Autodesk Inventor part; units mm, degrees
(part 2 of 3)
  spline S290 degree 2 poles (47.4504, -3.8325) (47.4504, -4.6086) (47.1983, -5.9037) (46.9314, -6.3684) knots 0 0 0 1 2 2 2
  spline S291 degree 2 poles (46.9314, -6.3684) (46.6595, -6.838) (45.8438, -7.3422) (45.2506, -7.3422) knots 0 0 0 1 2 2 2
  spline S292 degree 2 poles (45.2506, -7.3422) (45.048, -7.3422) (44.613, -7.2681) (44.5438, -7.2384) knots 0 0 0 1 2 2 2
  line L295 (44.5438, -7.2384) -> (44.5438, -6.0421)
  line L296 (44.5438, -6.0421) -> (44.6278, -6.0421)
  spline S293 degree 2 poles (44.6278, -6.0421) (44.7069, -6.1015) (45.0035, -6.23) (45.2605, -6.23) knots 0 0 0 1 2 2 2
  spline S294 degree 2 poles (45.2605, -6.23) (45.4731, -6.23) (45.8587, -6.0718) (46.002, -5.8988) knots 0 0 0 1 2 2 2
  spline S295 degree 2 poles (46.002, -5.8988) (46.1454, -5.7159) (46.3431, -5.1771) (46.3777, -4.7717) knots 0 0 0 1 2 2 2
  spline S296 degree 2 poles (46.3777, -4.7717) (46.1454, -4.9744) (45.7549, -5.1919) (45.4632, -5.1919) knots 0 0 0 1 2 2 2
  spline S297 degree 2 poles (45.4632, -5.1919) (45.2408, -5.1919) (44.8354, -5.0238) (44.6723, -4.8459) knots 0 0 0 1 2 2 2
  spline S298 degree 2 poles (44.6723, -4.8459) (44.4498, -4.6036) (44.1928, -3.8276) (44.1928, -3.2146) knots 0 0 0 1 2 2 2
  spline S299 degree 2 poles (44.1928, -3.2146) (44.1928, -2.7351) (44.4202, -1.9293) (44.6278, -1.6327) knots 0 0 0 1 2 2 2
  spline S300 degree 2 poles (44.6278, -1.6327) (44.8354, -1.3361) (45.4335, -1) (45.8043, -1) knots 0 0 0 1 2 2 2
  spline S301 degree 2 poles (45.8043, -1) (46.175, -1) (46.7534, -1.2966) (46.961, -1.608) knots 0 0 0 1 2 2 2
  spline S302 degree 2 poles (46.961, -1.608) (47.2032, -1.9541) (47.4504, -3.0515) (47.4504, -3.8325) knots 0 0 0 1 2 2 2
  spline S303 degree 2 poles (46.3925, -3.6051) (46.3925, -3.1058) (46.2739, -2.4632) (46.1701, -2.2853) knots 0 0 0 1 2 2 2
  spline S304 degree 2 poles (46.1701, -2.2853) (46.0959, -2.1518) (45.9081, -2.0381) (45.7994, -2.0381) knots 0 0 0 1 2 2 2
  spline S305 degree 2 poles (45.7994, -2.0381) (45.7054, -2.0381) (45.5275, -2.1468) (45.4434, -2.2853) knots 0 0 0 1 2 2 2
  spline S306 degree 2 poles (45.4434, -2.2853) (45.3693, -2.4039) (45.2655, -2.8636) (45.2655, -3.1355) knots 0 0 0 1 2 2 2
  spline S307 degree 2 poles (45.2655, -3.1355) (45.2655, -3.4321) (45.3693, -3.8127) (45.4632, -3.9264) knots 0 0 0 1 2 2 2
  spline S308 degree 2 poles (45.4632, -3.9264) (45.5522, -4.0401) (45.7895, -4.1291) (45.9328, -4.1291) knots 0 0 0 1 2 2 2
  spline S309 degree 2 poles (45.9328, -4.1291) (46.0515, -4.1291) (46.3085, -4.0352) (46.3827, -3.9857) knots 0 0 0 1 2 2 2
  spline S310 degree 2 poles (46.3827, -3.9857) (46.3827, -3.9412) (46.3925, -3.7732) (46.3925, -3.6051) knots 0 0 0 1 2 2 2
  line L297 (43.6441, 12.8852) -> (40.8264, 12.8852)
  line L298 (40.8264, 12.8852) -> (40.8264, 13.948)
  line L299 (40.8264, 13.948) -> (41.7261, 13.948)
  line L300 (41.7261, 13.948) -> (41.7261, 17.1759)
  line L301 (41.7261, 17.1759) -> (40.8264, 17.1759)
  line L302 (40.8264, 17.1759) -> (40.8264, 18.1695)
  spline S311 degree 2 poles (40.8264, 18.1695) (41.0241, 18.1695) (41.4147, 18.2437) (41.5333, 18.3228) knots 0 0 0 1 2 2 2
  spline S312 degree 2 poles (41.5333, 18.3228) (41.6668, 18.4216) (41.82, 18.7528) (41.8299, 19) knots 0 0 0 1 2 2 2
  line L303 (41.8299, 19) -> (42.7642, 19)
  line L304 (42.7642, 19) -> (42.7642, 13.948)
  line L305 (42.7642, 13.948) -> (43.6441, 13.948)
  line L306 (43.6441, 13.948) -> (43.6441, 12.8852)
  line L307 (47.4702, 17.7741) -> (45.656, 12.8852)
  line L308 (45.656, 12.8852) -> (44.4647, 12.8852)
  line L309 (44.4647, 12.8852) -> (46.3678, 17.8334)
  line L310 (46.3678, 17.8334) -> (44.3361, 17.8334)
  line L311 (44.3361, 17.8334) -> (44.3361, 18.9852)
  line L312 (44.3361, 18.9852) -> (47.4702, 18.9852)
  line L313 (47.4702, 18.9852) -> (47.4702, 17.7741)
  line L314 (23.6441, 12.8852) -> (20.8264, 12.8852)
  line L315 (20.8264, 12.8852) -> (20.8264, 13.948)
  line L316 (20.8264, 13.948) -> (21.7261, 13.948)
  line L317 (21.7261, 13.948) -> (21.7261, 17.1759)
  line L318 (21.7261, 17.1759) -> (20.8264, 17.1759)
  line L319 (20.8264, 17.1759) -> (20.8264, 18.1695)
  spline S313 degree 2 poles (20.8264, 18.1695) (21.0241, 18.1695) (21.4147, 18.2437) (21.5333, 18.3228) knots 0 0 0 1 2 2 2
  spline S314 degree 2 poles (21.5333, 18.3228) (21.6668, 18.4216) (21.82, 18.7528) (21.8299, 19) knots 0 0 0 1 2 2 2
  line L320 (21.8299, 19) -> (22.7642, 19)
  line L321 (22.7642, 19) -> (22.7642, 13.948)
  line L322 (22.7642, 13.948) -> (23.6441, 13.948)
  line L323 (23.6441, 13.948) -> (23.6441, 12.8852)
  spline S315 degree 2 poles (27.4652, 14.9515) (27.4652, 14.472) (27.2378, 13.6613) (27.0154, 13.3696) knots 0 0 0 1 2 2 2
  spline S316 degree 2 poles (27.0154, 13.3696) (26.7929, 13.078) (26.175, 12.7566) (25.7252, 12.7566) knots 0 0 0 1 2 2 2
  spline S317 degree 2 poles (25.7252, 12.7566) (25.2506, 12.7616) (24.5685, 12.984) (24.346, 13.1274) knots 0 0 0 1 2 2 2
  line L324 (24.346, 13.1274) -> (24.346, 14.4571)
  line L325 (24.346, 14.4571) -> (24.4449, 14.4571)
  spline S318 degree 2 poles (24.4449, 14.4571) (24.524, 14.3929) (24.7217, 14.2248) (24.8848, 14.1358) knots 0 0 0 1 2 2 2
  spline S319 degree 2 poles (24.8848, 14.1358) (25.0381, 14.0518) (25.3495, 13.9381) (25.5423, 13.9381) knots 0 0 0 1 2 2 2
  spline S320 degree 2 poles (25.5423, 13.9381) (25.7104, 13.9381) (26.091, 14.0567) (26.2096, 14.2149) knots 0 0 0 1 2 2 2
  spline S321 degree 2 poles (26.2096, 14.2149) (26.2937, 14.3385) (26.3925, 14.64) (26.3925, 14.8921) knots 0 0 0 1 2 2 2
  spline S322 degree 2 poles (26.3925, 14.8921) (26.3925, 15.1096) (26.269, 15.4161) (26.1701, 15.51) knots 0 0 0 1 2 2 2
  spline S323 degree 2 poles (26.1701, 15.51) (26.0218, 15.6485) (25.6115, 15.7276) (25.4632, 15.7276) knots 0 0 0 1 2 2 2
  spline S324 degree 2 poles (25.4632, 15.7276) (25.2259, 15.7276) (24.786, 15.6188) (24.6229, 15.5595) knots 0 0 0 1 2 2 2
  line L326 (24.6229, 15.5595) -> (24.5289, 15.5595)
  line L327 (24.5289, 15.5595) -> (24.5289, 18.9852)
  line L328 (24.5289, 18.9852) -> (27.3466, 18.9852)
  line L329 (27.3466, 18.9852) -> (27.3466, 17.8334)
  line L330 (27.3466, 17.8334) -> (25.5374, 17.8334)
  line L331 (25.5374, 17.8334) -> (25.5374, 16.82)
  spline S325 degree 2 poles (25.5374, 16.82) (25.6214, 16.8299) (25.8587, 16.8398) (25.9279, 16.8398) knots 0 0 0 1 2 2 2
  spline S326 degree 2 poles (25.9279, 16.8398) (26.2344, 16.8398) (26.7534, 16.6618) (26.9511, 16.4789) knots 0 0 0 1 2 2 2
  spline S327 degree 2 poles (26.9511, 16.4789) (27.1983, 16.2515) (27.4652, 15.4952) (27.4652, 14.9515) knots 0 0 0 1 2 2 2
  line L332 (33.6441, 12.7863) -> (30.8264, 12.7863)
  line L333 (30.8264, 12.7863) -> (30.8264, 13.8491)
  line L334 (30.8264, 13.8491) -> (31.7261, 13.8491)
  line L335 (31.7261, 13.8491) -> (31.7261, 17.0771)
  line L336 (31.7261, 17.0771) -> (30.8264, 17.0771)
  line L337 (30.8264, 17.0771) -> (30.8264, 18.0707)
  spline S328 degree 2 poles (30.8264, 18.0707) (31.0241, 18.0707) (31.4147, 18.1448) (31.5333, 18.2239) knots 0 0 0 1 2 2 2
  spline S329 degree 2 poles (31.5333, 18.2239) (31.6668, 18.3228) (31.82, 18.654) (31.8299, 18.9011) knots 0 0 0 1 2 2 2
  line L338 (31.8299, 18.9011) -> (32.7642, 18.9011)
  line L339 (32.7642, 18.9011) -> (32.7642, 13.8491)
  line L340 (32.7642, 13.8491) -> (33.6441, 13.8491)
  line L341 (33.6441, 13.8491) -> (33.6441, 12.7863)
  spline S330 degree 2 poles (37.5394, 14.8625) (37.5394, 13.8985) (36.6842, 12.6578) (35.9427, 12.6578) knots 0 0 0 1 2 2 2
  spline S331 degree 2 poles (35.9427, 12.6578) (35.572, 12.6578) (34.9837, 12.9643) (34.781, 13.2658) knots 0 0 0 1 2 2 2
  spline S332 degree 2 poles (34.781, 13.2658) (34.5388, 13.6168) (34.2818, 14.729) (34.2818, 15.5051) knots 0 0 0 1 2 2 2
  spline S333 degree 2 poles (34.2818, 15.5051) (34.2818, 16.3059) (34.524, 17.5516) (34.7959, 18.0311) knots 0 0 0 1 2 2 2
  spline S334 degree 2 poles (34.7959, 18.0311) (35.0529, 18.4859) (35.8982, 19) (36.4716, 19) knots 0 0 0 1 2 2 2
  spline S335 degree 2 poles (36.4716, 19) (36.6793, 19) (37.0994, 18.9209) (37.1785, 18.8962) knots 0 0 0 1 2 2 2
  line L342 (37.1785, 18.8962) -> (37.1785, 17.6999)
  line L343 (37.1785, 17.6999) -> (37.0994, 17.6999)
  spline S336 degree 2 poles (37.0994, 17.6999) (37.0253, 17.7543) (36.6842, 17.8878) (36.4618, 17.8878) knots 0 0 0 1 2 2 2
  spline S337 degree 2 poles (36.4618, 17.8878) (35.9625, 17.8878) (35.4187, 17.1314) (35.3545, 16.4295) knots 0 0 0 1 2 2 2
  spline S338 degree 2 poles (35.3545, 16.4295) (35.567, 16.6223) (35.9971, 16.8497) (36.269, 16.8497) knots 0 0 0 1 2 2 2
  spline S339 degree 2 poles (36.269, 16.8497) (36.4964, 16.8497) (36.9017, 16.6717) (37.0599, 16.5036) knots 0 0 0 1 2 2 2
  spline S340 degree 2 poles (37.0599, 16.5036) (37.2774, 16.2614) (37.5394, 15.4754) (37.5394, 14.8625) knots 0 0 0 1 2 2 2
  spline S341 degree 2 poles (36.2937, 13.943) (36.3777, 14.0913) (36.4667, 14.4374) (36.4667, 14.7883) knots 0 0 0 1 2 2 2
  spline S342 degree 2 poles (36.4667, 14.7883) (36.4667, 15.0849) (36.3629, 15.4705) (36.269, 15.5842) knots 0 0 0 1 2 2 2
  spline S343 degree 2 poles (36.269, 15.5842) (36.175, 15.7028) (35.9378, 15.7869) (35.7994, 15.7869) knots 0 0 0 1 2 2 2
  spline S344 degree 2 poles (35.7994, 15.7869) (35.6906, 15.7869) (35.4533, 15.7028) (35.3495, 15.6435) knots 0 0 0 1 2 2 2
  spline S345 degree 2 poles (35.3495, 15.6435) (35.3495, 15.604) (35.3446, 15.4161) (35.3446, 15.2728) knots 0 0 0 1 2 2 2
  spline S346 degree 2 poles (35.3446, 15.2728) (35.3446, 14.7438) (35.4731, 14.1062) (35.572, 13.943) knots 0 0 0 1 2 2 2
  spline S347 degree 2 poles (35.572, 13.943) (35.6461, 13.8096) (35.834, 13.6959) (35.9427, 13.6959) knots 0 0 0 1 2 2 2
  spline S348 degree 2 poles (35.9427, 13.6959) (36.0267, 13.6959) (36.2245, 13.8194) (36.2937, 13.943) knots 0 0 0 1 2 2 2
  line L344 (23.8319, -7.2186) -> (20.6979, -7.2186)
  line L345 (20.6979, -7.2186) -> (20.6979, -6.225)
  spline S349 degree 2 poles (20.6979, -6.225) (21.0983, -5.7703) (21.7261, -4.9694) (21.9683, -4.6086) knots 0 0 0 1 2 2 2
  spline S350 degree 2 poles (21.9683, -4.6086) (22.2797, -4.139) (22.5615, -3.4222) (22.5615, -3.0465) knots 0 0 0 1 2 2 2
  spline S351 degree 2 poles (22.5615, -3.0465) (22.5615, -2.6214) (22.2056, -2.1666) (21.8892, -2.1666) knots 0 0 0 1 2 2 2
  spline S352 degree 2 poles (21.8892, -2.1666) (21.7261, -2.1666) (21.4394, -2.2803) (21.2861, -2.3693) knots 0 0 0 1 2 2 2
  spline S353 degree 2 poles (21.2861, -2.3693) (21.1428, -2.4632) (20.9352, -2.6609) (20.8857, -2.7104) knots 0 0 0 1 2 2 2
  line L346 (20.8857, -2.7104) -> (20.8017, -2.7104)
  line L347 (20.8017, -2.7104) -> (20.8017, -1.3806)
  spline S354 degree 2 poles (20.8017, -1.3806) (20.9797, -1.257) (21.7508, -1) (22.1018, -1) knots 0 0 0 1 2 2 2
  spline S355 degree 2 poles (22.1018, -1) (22.863, -1) (23.6441, -1.9689) (23.6441, -2.8438) knots 0 0 0 1 2 2 2
  spline S356 degree 2 poles (23.6441, -2.8438) (23.6441, -3.3827) (23.2882, -4.4207) (22.8779, -5.0139) knots 0 0 0 1 2 2 2
  spline S357 degree 2 poles (22.8779, -5.0139) (22.6208, -5.3797) (22.1314, -5.9482) (22.0227, -6.0669) knots 0 0 0 1 2 2 2
  line L348 (22.0227, -6.0669) -> (23.8319, -6.0669)
  line L349 (23.8319, -6.0669) -> (23.8319, -7.2186)
  line L350 (27.4702, -2.3297) -> (25.656, -7.2186)
  line L351 (25.656, -7.2186) -> (24.4647, -7.2186)
  line L352 (24.4647, -7.2186) -> (26.3678, -2.2704)
  line L353 (26.3678, -2.2704) -> (24.3361, -2.2704)
  line L354 (24.3361, -2.2704) -> (24.3361, -1.1186)
  line L355 (24.3361, -1.1186) -> (27.4702, -1.1186)
  line L356 (27.4702, -1.1186) -> (27.4702, -2.3297)
  line L357 (23.8319, 2.7814) -> (20.6979, 2.7814)
  line L358 (20.6979, 2.7814) -> (20.6979, 3.775)
  spline S358 degree 2 poles (20.6979, 3.775) (21.0983, 4.2297) (21.7261, 5.0306) (21.9683, 5.3914) knots 0 0 0 1 2 2 2
  spline S359 degree 2 poles (21.9683, 5.3914) (22.2797, 5.861) (22.5615, 6.5778) (22.5615, 6.9535) knots 0 0 0 1 2 2 2
  spline S360 degree 2 poles (22.5615, 6.9535) (22.5615, 7.3786) (22.2056, 7.8334) (21.8892, 7.8334) knots 0 0 0 1 2 2 2
  spline S361 degree 2 poles (21.8892, 7.8334) (21.7261, 7.8334) (21.4394, 7.7197) (21.2861, 7.6307) knots 0 0 0 1 2 2 2
  spline S362 degree 2 poles (21.2861, 7.6307) (21.1428, 7.5368) (20.9352, 7.3391) (20.8857, 7.2896) knots 0 0 0 1 2 2 2
  line L359 (20.8857, 7.2896) -> (20.8017, 7.2896)
  line L360 (20.8017, 7.2896) -> (20.8017, 8.6194)
  spline S363 degree 2 poles (20.8017, 8.6194) (20.9797, 8.743) (21.7508, 9) (22.1018, 9) knots 0 0 0 1 2 2 2
  spline S364 degree 2 poles (22.1018, 9) (22.863, 9) (23.6441, 8.0311) (23.6441, 7.1562) knots 0 0 0 1 2 2 2
  spline S365 degree 2 poles (23.6441, 7.1562) (23.6441, 6.6173) (23.2882, 5.5793) (22.8779, 4.9861) knots 0 0 0 1 2 2 2
  spline S366 degree 2 poles (22.8779, 4.9861) (22.6208, 4.6203) (22.1314, 4.0518) (22.0227, 3.9331) knots 0 0 0 1 2 2 2
  line L361 (22.0227, 3.9331) -> (23.8319, 3.9331)
  line L362 (23.8319, 3.9331) -> (23.8319, 2.7814)
  line L363 (27.3763, 2.7814) -> (24.5586, 2.7814)
  line L364 (24.5586, 2.7814) -> (24.5586, 3.8442)
  line L365 (24.5586, 3.8442) -> (25.4583, 3.8442)
  line L366 (25.4583, 3.8442) -> (25.4583, 7.0721)
  line L367 (25.4583, 7.0721) -> (24.5586, 7.0721)
  line L368 (24.5586, 7.0721) -> (24.5586, 8.0657)
  spline S367 degree 2 poles (24.5586, 8.0657) (24.7563, 8.0657) (25.1468, 8.1399) (25.2655, 8.219) knots 0 0 0 1 2 2 2
  spline S368 degree 2 poles (25.2655, 8.219) (25.3989, 8.3178) (25.5522, 8.649) (25.5621, 8.8962) knots 0 0 0 1 2 2 2
  line L369 (25.5621, 8.8962) -> (26.4964, 8.8962)
  line L370 (26.4964, 8.8962) -> (26.4964, 3.8442)
  line L371 (26.4964, 3.8442) -> (27.3763, 3.8442)
  line L372 (27.3763, 3.8442) -> (27.3763, 2.7814)
  line L373 (53.8319, 2.7814) -> (50.6979, 2.7814)
  line L374 (50.6979, 2.7814) -> (50.6979, 3.775)
  spline S369 degree 2 poles (50.6979, 3.775) (51.0983, 4.2297) (51.7261, 5.0306) (51.9683, 5.3914) knots 0 0 0 1 2 2 2
  spline S370 degree 2 poles (51.9683, 5.3914) (52.2797, 5.861) (52.5615, 6.5778) (52.5615, 6.9535) knots 0 0 0 1 2 2 2
  spline S371 degree 2 poles (52.5615, 6.9535) (52.5615, 7.3786) (52.2056, 7.8334) (51.8892, 7.8334) knots 0 0 0 1 2 2 2
  spline S372 degree 2 poles (51.8892, 7.8334) (51.7261, 7.8334) (51.4394, 7.7197) (51.2861, 7.6307) knots 0 0 0 1 2 2 2
  spline S373 degree 2 poles (51.2861, 7.6307) (51.1428, 7.5368) (50.9352, 7.3391) (50.8857, 7.2896) knots 0 0 0 1 2 2 2
  line L375 (50.8857, 7.2896) -> (50.8017, 7.2896)
  line L376 (50.8017, 7.2896) -> (50.8017, 8.6194)
  spline S374 degree 2 poles (50.8017, 8.6194) (50.9797, 8.743) (51.7508, 9) (52.1018, 9) knots 0 0 0 1 2 2 2
  spline S375 degree 2 poles (52.1018, 9) (52.863, 9) (53.6441, 8.0311) (53.6441, 7.1562) knots 0 0 0 1 2 2 2
  spline S376 degree 2 poles (53.6441, 7.1562) (53.6441, 6.6173) (53.2882, 5.5793) (52.8779, 4.9861) knots 0 0 0 1 2 2 2
  spline S377 degree 2 poles (52.8779, 4.9861) (52.6208, 4.6203) (52.1314, 4.0518) (52.0227, 3.9331) knots 0 0 0 1 2 2 2
  line L377 (52.0227, 3.9331) -> (53.8319, 3.9331)
  line L378 (53.8319, 3.9331) -> (53.8319, 2.7814)
  line L379 (57.6086, 4.205) -> (57.0352, 4.205)
  line L380 (57.0352, 4.205) -> (57.0352, 2.7665)
  line L381 (57.0352, 2.7665) -> (55.9971, 2.7665)
  line L382 (55.9971, 2.7665) -> (55.9971, 4.205)
  line L383 (55.9971, 4.205) -> (54.1285, 4.205)
  line L384 (54.1285, 4.205) -> (54.1285, 5.342)
  line L385 (54.1285, 5.342) -> (55.9625, 8.8814)
  line L386 (55.9625, 8.8814) -> (57.0352, 8.8814)
  line L387 (57.0352, 8.8814) -> (57.0352, 5.3024)
  line L388 (57.0352, 5.3024) -> (57.6086, 5.3024)
  line L389 (57.6086, 5.3024) -> (57.6086, 4.205)
  line L390 (55.9971, 5.3024) -> (55.9971, 7.3737)
  line L391 (55.9971, 7.3737) -> (54.9244, 5.3024)
  line L392 (54.9244, 5.3024) -> (55.9971, 5.3024)
  line L393 (43.8319, 2.7715) -> (40.6979, 2.7715)
  line L394 (40.6979, 2.7715) -> (40.6979, 3.7651)
  spline S378 degree 2 poles (40.6979, 3.7651) (41.0983, 4.2199) (41.7261, 5.0207) (41.9683, 5.3815) knots 0 0 0 1 2 2 2
  spline S379 degree 2 poles (41.9683, 5.3815) (42.2797, 5.8511) (42.5615, 6.5679) (42.5615, 6.9436) knots 0 0 0 1 2 2 2
  spline S380 degree 2 poles (42.5615, 6.9436) (42.5615, 7.3687) (42.2056, 7.8235) (41.8892, 7.8235) knots 0 0 0 1 2 2 2
  spline S381 degree 2 poles (41.8892, 7.8235) (41.7261, 7.8235) (41.4394, 7.7098) (41.2861, 7.6208) knots 0 0 0 1 2 2 2
  spline S382 degree 2 poles (41.2861, 7.6208) (41.1428, 7.5269) (40.9352, 7.3292) (40.8857, 7.2797) knots 0 0 0 1 2 2 2
  line L395 (40.8857, 7.2797) -> (40.8017, 7.2797)
  line L396 (40.8017, 7.2797) -> (40.8017, 8.6095)
  spline S383 degree 2 poles (40.8017, 8.6095) (40.9797, 8.7331) (41.7508, 8.9901) (42.1018, 8.9901) knots 0 0 0 1 2 2 2
  spline S384 degree 2 poles (42.1018, 8.9901) (42.863, 8.9901) (43.6441, 8.0212) (43.6441, 7.1463) knots 0 0 0 1 2 2 2
  spline S385 degree 2 poles (43.6441, 7.1463) (43.6441, 6.6075) (43.2882, 5.5694) (42.8779, 4.9762) knots 0 0 0 1 2 2 2
  spline S386 degree 2 poles (42.8779, 4.9762) (42.6208, 4.6104) (42.1314, 4.0419) (42.0227, 3.9233) knots 0 0 0 1 2 2 2
  line L397 (42.0227, 3.9233) -> (43.8319, 3.9233)
  line L398 (43.8319, 3.9233) -> (43.8319, 2.7715)
  spline S387 degree 2 poles (47.4553, 4.6203) (47.4553, 4.1704) (47.223, 3.4339) (47.0006, 3.1768) knots 0 0 0 1 2 2 2
  spline S388 degree 2 poles (47.0006, 3.1768) (46.7732, 2.9198) (46.1652, 2.6429) (45.7301, 2.6429) knots 0 0 0 1 2 2 2
  spline S389 degree 2 poles (45.7301, 2.6429) (45.2309, 2.6429) (44.519, 2.8802) (44.2966, 3.0285) knots 0 0 0 1 2 2 2
  line L399 (44.2966, 3.0285) -> (44.2966, 4.3533)
  line L400 (44.2966, 4.3533) -> (44.4004, 4.3533)
  spline S390 degree 2 poles (44.4004, 4.3533) (44.6327, 4.1408) (45.2655, 3.8244) (45.5275, 3.8244) knots 0 0 0 1 2 2 2
  spline S391 degree 2 poles (45.5275, 3.8244) (45.6807, 3.8244) (46.0465, 3.9035) (46.1701, 4.032) knots 0 0 0 1 2 2 2
  spline S392 degree 2 poles (46.1701, 4.032) (46.264, 4.1358) (46.3827, 4.4374) (46.3827, 4.7092) knots 0 0 0 1 2 2 2
  spline S393 degree 2 poles (46.3827, 4.7092) (46.3827, 4.9811) (46.2146, 5.2728) (46.0811, 5.342) knots 0 0 0 1 2 2 2
  spline S394 degree 2 poles (46.0811, 5.342) (45.9427, 5.4112) (45.5571, 5.426) (45.4138, 5.426) knots 0 0 0 1 2 2 2
  line L401 (45.4138, 5.426) -> (45.2309, 5.426)
  line L402 (45.2309, 5.426) -> (45.2309, 6.4987)
  line L403 (45.2309, 6.4987) -> (45.3989, 6.4987)
  spline S395 degree 2 poles (45.3989, 6.4987) (45.5917, 6.4987) (45.913, 6.5481) (46.0267, 6.6223) knots 0 0 0 1 2 2 2
  spline S396 degree 2 poles (46.0267, 6.6223) (46.1404, 6.7014) (46.269, 6.9782) (46.269, 7.2155) knots 0 0 0 1 2 2 2
  spline S397 degree 2 poles (46.269, 7.2155) (46.269, 7.4033) (46.1503, 7.6357) (46.0613, 7.6999) knots 0 0 0 1 2 2 2
  spline S398 degree 2 poles (46.0613, 7.6999) (45.9575, 7.7741) (45.6857, 7.8235) (45.5868, 7.8235) knots 0 0 0 1 2 2 2
  spline S399 degree 2 poles (45.5868, 7.8235) (45.4335, 7.8235) (45.1073, 7.7197) (44.9541, 7.6357) knots 0 0 0 1 2 2 2
  spline S400 degree 2 poles (44.9541, 7.6357) (44.8354, 7.5714) (44.5734, 7.3638) (44.5092, 7.3094) knots 0 0 0 1 2 2 2
  line L404 (44.5092, 7.3094) -> (44.4202, 7.3094)
  line L405 (44.4202, 7.3094) -> (44.4202, 8.6144)
  spline S401 degree 2 poles (44.4202, 8.6144) (44.6377, 8.7479) (45.3841, 9) (45.7746, 9) knots 0 0 0 1 2 2 2
  spline S402 degree 2 poles (45.7746, 9) (46.1553, 9) (46.7089, 8.8122) (46.9066, 8.6293) knots 0 0 0 1 2 2 2
  spline S403 degree 2 poles (46.9066, 8.6293) (47.1241, 8.4365) (47.3417, 7.8433) (47.3417, 7.4725) knots 0 0 0 1 2 2 2
  spline S404 degree 2 poles (47.3417, 7.4725) (47.3417, 6.9485) (46.9215, 6.1675) (46.5804, 6.0538) knots 0 0 0 1 2 2 2
  line L406 (46.5804, 6.0538) -> (46.5804, 5.9945)
  spline S405 degree 2 poles (46.5804, 5.9945) (46.7336, 5.9648) (47.0203, 5.8066) (47.1588, 5.6287) knots 0 0 0 1 2 2 2
  spline S406 degree 2 poles (47.1588, 5.6287) (47.2873, 5.4705) (47.4553, 4.9663) (47.4553, 4.6203) knots 0 0 0 1 2 2 2
  line L407 (53.6441, 12.7616) -> (50.8264, 12.7616)
  line L408 (50.8264, 12.7616) -> (50.8264, 13.8244)
  line L409 (50.8264, 13.8244) -> (51.7261, 13.8244)
  line L410 (51.7261, 13.8244) -> (51.7261, 17.0524)
  line L411 (51.7261, 17.0524) -> (50.8264, 17.0524)
  line L412 (50.8264, 17.0524) -> (50.8264, 18.0459)
  spline S407 degree 2 poles (50.8264, 18.0459) (51.0241, 18.0459) (51.4147, 18.1201) (51.5333, 18.1992) knots 0 0 0 1 2 2 2
  spline S408 degree 2 poles (51.5333, 18.1992) (51.6668, 18.2981) (51.82, 18.6293) (51.8299, 18.8764) knots 0 0 0 1 2 2 2
  line L413 (51.8299, 18.8764) -> (52.7642, 18.8764)
  line L414 (52.7642, 18.8764) -> (52.7642, 13.8244)
  line L415 (52.7642, 13.8244) -> (53.6441, 13.8244)
  line L416 (53.6441, 13.8244) -> (53.6441, 12.7616)
  spline S409 degree 2 poles (57.5542, 14.4571) (57.5542, 14.0666) (57.3268, 13.3894) (57.1093, 13.1422) knots 0 0 0 1 2 2 2
  spline S410 degree 2 poles (57.1093, 13.1422) (56.8918, 12.8951) (56.264, 12.6182) (55.8587, 12.6182) knots 0 0 0 1 2 2 2
  spline S411 degree 2 poles (55.8587, 12.6182) (55.4286, 12.6182) (54.781, 12.9) (54.5784, 13.1422) knots 0 0 0 1 2 2 2
  spline S412 degree 2 poles (54.5784, 13.1422) (54.3707, 13.3844) (54.178, 14.0419) (54.178, 14.4077) knots 0 0 0 1 2 2 2
  spline S413 degree 2 poles (54.178, 14.4077) (54.178, 14.9317) (54.5833, 15.6287) (54.9639, 15.861) knots 0 0 0 1 2 2 2
  line L417 (54.9639, 15.861) -> (54.9639, 15.8857)
  spline S414 degree 2 poles (54.9639, 15.8857) (54.5882, 16.1477) (54.2917, 16.8942) (54.2917, 17.3539) knots 0 0 0 1 2 2 2
  spline S415 degree 2 poles (54.2917, 17.3539) (54.2917, 17.69) (54.4993, 18.2783) (54.7069, 18.5106) knots 0 0 0 1 2 2 2
  spline S416 degree 2 poles (54.7069, 18.5106) (54.8997, 18.7331) (55.4978, 19) (55.8735, 19) knots 0 0 0 1 2 2 2
  spline S417 degree 2 poles (55.8735, 19) (56.269, 19) (56.8572, 18.7578) (57.0451, 18.56) knots 0 0 0 1 2 2 2
  spline S418 degree 2 poles (57.0451, 18.56) (57.2378, 18.3623) (57.4455, 17.7889) (57.4455, 17.4577) knots 0 0 0 1 2 2 2
  spline S419 degree 2 poles (57.4455, 17.4577) (57.4455, 17.0227) (57.0945, 16.3257) (56.7287, 16.0835) knots 0 0 0 1 2 2 2
  line L418 (56.7287, 16.0835) -> (56.7287, 16.0637)
  spline S420 degree 2 poles (56.7287, 16.0637) (57.1538, 15.8165) (57.5542, 15.0157) (57.5542, 14.4571) knots 0 0 0 1 2 2 2
  spline S421 degree 2 poles (56.4964, 14.3929) (56.4964, 14.6944) (56.3184, 15.0108) (56.0218, 15.2135) knots 0 0 0 1 2 2 2
  spline S422 degree 2 poles (56.0218, 15.2135) (55.9378, 15.2678) (55.6263, 15.4408) (55.5028, 15.515) knots 0 0 0 1 2 2 2
  spline S423 degree 2 poles (55.5028, 15.515) (55.394, 15.3568) (55.216, 14.8823) (55.216, 14.6005) knots 0 0 0 1 2 2 2
  spline S424 degree 2 poles (55.216, 14.6005) (55.216, 14.1754) (55.5967, 13.6662) (55.9081, 13.6662) knots 0 0 0 1 2 2 2
  spline S425 degree 2 poles (55.9081, 13.6662) (55.9921, 13.6662) (56.2096, 13.7453) (56.2937, 13.8244) knots 0 0 0 1 2 2 2
  spline S426 degree 2 poles (56.2937, 13.8244) (56.3827, 13.9183) (56.4964, 14.1754) (56.4964, 14.3929) knots 0 0 0 1 2 2 2
  spline S427 degree 2 poles (56.4074, 17.2797) (56.4074, 17.5912) (56.1207, 17.9619) (55.8735, 17.9619) knots 0 0 0 1 2 2 2
  spline S428 degree 2 poles (55.8735, 17.9619) (55.6412, 17.9619) (55.3495, 17.6258) (55.3495, 17.3786) knots 0 0 0 1 2 2 2
  spline S429 degree 2 poles (55.3495, 17.3786) (55.3495, 17.1364) (55.5225, 16.8348) (55.7104, 16.7113) knots 0 0 0 1 2 2 2
  spline S430 degree 2 poles (55.7104, 16.7113) (55.7895, 16.6519) (56.007, 16.5284) (56.1948, 16.4295) knots 0 0 0 1 2 2 2
  spline S431 degree 2 poles (56.1948, 16.4295) (56.3036, 16.6371) (56.4074, 17.0276) (56.4074, 17.2797) knots 0 0 0 1 2 2 2
  line L419 (33.8319, -7.2384) -> (30.6979, -7.2384)
  line L420 (30.6979, -7.2384) -> (30.6979, -6.2448)
  spline S432 degree 2 poles (30.6979, -6.2448) (31.0983, -5.79) (31.7261, -4.9892) (31.9683, -4.6284) knots 0 0 0 1 2 2 2
  spline S433 degree 2 poles (31.9683, -4.6284) (32.2797, -4.1588) (32.5615, -3.442) (32.5615, -3.0663) knots 0 0 0 1 2 2 2
  spline S434 degree 2 poles (32.5615, -3.0663) (32.5615, -2.6412) (32.2056, -2.1864) (31.8892, -2.1864) knots 0 0 0 1 2 2 2
  spline S435 degree 2 poles (31.8892, -2.1864) (31.7261, -2.1864) (31.4394, -2.3001) (31.2861, -2.3891) knots 0 0 0 1 2 2 2
  spline S436 degree 2 poles (31.2861, -2.3891) (31.1428, -2.483) (30.9352, -2.6807) (30.8857, -2.7301) knots 0 0 0 1 2 2 2
  line L421 (30.8857, -2.7301) -> (30.8017, -2.7301)
  line L422 (30.8017, -2.7301) -> (30.8017, -1.4004)
  spline S437 degree 2 poles (30.8017, -1.4004) (30.9797, -1.2768) (31.7508, -1.0198) (32.1018, -1.0198) knots 0 0 0 1 2 2 2
  spline S438 degree 2 poles (32.1018, -1.0198) (32.863, -1.0198) (33.6441, -1.9887) (33.6441, -2.8636) knots 0 0 0 1 2 2 2
  spline S439 degree 2 poles (33.6441, -2.8636) (33.6441, -3.4024) (33.2882, -4.4405) (32.8779, -5.0337) knots 0 0 0 1 2 2 2
  spline S440 degree 2 poles (32.8779, -5.0337) (32.6208, -5.3995) (32.1314, -5.968) (32.0227, -6.0866) knots 0 0 0 1 2 2 2
  line L423 (32.0227, -6.0866) -> (33.8319, -6.0866)
  line L424 (33.8319, -6.0866) -> (33.8319, -7.2384)
  spline S441 degree 2 poles (37.5542, -5.5429) (37.5542, -5.9334) (37.3268, -6.6106) (37.1093, -6.8578) knots 0 0 0 1 2 2 2
  spline S442 degree 2 poles (37.1093, -6.8578) (36.8918, -7.1049) (36.264, -7.3818) (35.8587, -7.3818) knots 0 0 0 1 2 2 2
  spline S443 degree 2 poles (35.8587, -7.3818) (35.4286, -7.3818) (34.781, -7.1) (34.5784, -6.8578) knots 0 0 0 1 2 2 2
  spline S444 degree 2 poles (34.5784, -6.8578) (34.3707, -6.6156) (34.178, -5.9581) (34.178, -5.5923) knots 0 0 0 1 2 2 2
  spline S445 degree 2 poles (34.178, -5.5923) (34.178, -5.0683) (34.5833, -4.3713) (34.9639, -4.139) knots 0 0 0 1 2 2 2
  line L425 (34.9639, -4.139) -> (34.9639, -4.1143)
  spline S446 degree 2 poles (34.9639, -4.1143) (34.5882, -3.8523) (34.2917, -3.1058) (34.2917, -2.6461) knots 0 0 0 1 2 2 2
  spline S447 degree 2 poles (34.2917, -2.6461) (34.2917, -2.31) (34.4993, -1.7217) (34.7069, -1.4894) knots 0 0 0 1 2 2 2
  spline S448 degree 2 poles (34.7069, -1.4894) (34.8997, -1.2669) (35.4978, -1) (35.8735, -1) knots 0 0 0 1 2 2 2
  spline S449 degree 2 poles (35.8735, -1) (36.269, -1) (36.8572, -1.2422) (37.0451, -1.44) knots 0 0 0 1 2 2 2
  spline S450 degree 2 poles (37.0451, -1.44) (37.2378, -1.6377) (37.4455, -2.2111) (37.4455, -2.5423) knots 0 0 0 1 2 2 2
  spline S451 degree 2 poles (37.4455, -2.5423) (37.4455, -2.9773) (37.0945, -3.6743) (36.7287, -3.9165) knots 0 0 0 1 2 2 2
  line L426 (36.7287, -3.9165) -> (36.7287, -3.9363)
  spline S452 degree 2 poles (36.7287, -3.9363) (37.1538, -4.1835) (37.5542, -4.9843) (37.5542, -5.5429) knots 0 0 0 1 2 2 2
  spline S453 degree 2 poles (36.4964, -5.6071) (36.4964, -5.3056) (36.3184, -4.9892) (36.0218, -4.7865) knots 0 0 0 1 2 2 2
  spline S454 degree 2 poles (36.0218, -4.7865) (35.9378, -4.7322) (35.6263, -4.5592) (35.5028, -4.485) knots 0 0 0 1 2 2 2
  spline S455 degree 2 poles (35.5028, -4.485) (35.394, -4.6432) (35.216, -5.1177) (35.216, -5.3995) knots 0 0 0 1 2 2 2
  spline S456 degree 2 poles (35.216, -5.3995) (35.216, -5.8246) (35.5967, -6.3338) (35.9081, -6.3338) knots 0 0 0 1 2 2 2
  spline S457 degree 2 poles (35.9081, -6.3338) (35.9921, -6.3338) (36.2096, -6.2547) (36.2937, -6.1756) knots 0 0 0 1 2 2 2
  spline S458 degree 2 poles (36.2937, -6.1756) (36.3827, -6.0817) (36.4964, -5.8246) (36.4964, -5.6071) knots 0 0 0 1 2 2 2
  spline S459 degree 2 poles (36.4074, -2.7203) (36.4074, -2.4088) (36.1207, -2.0381) (35.8735, -2.0381) knots 0 0 0 1 2 2 2
  spline S460 degree 2 poles (35.8735, -2.0381) (35.6412, -2.0381) (35.3495, -2.3742) (35.3495, -2.6214) knots 0 0 0 1 2 2 2
  spline S461 degree 2 poles (35.3495, -2.6214) (35.3495, -2.8636) (35.5225, -3.1652) (35.7104, -3.2887) knots 0 0 0 1 2 2 2
  spline S462 degree 2 poles (35.7104, -3.2887) (35.7895, -3.3481) (36.007, -3.4716) (36.1948, -3.5705) knots 0 0 0 1 2 2 2
  spline S463 degree 2 poles (36.1948, -3.5705) (36.3036, -3.3629) (36.4074, -2.9724) (36.4074, -2.7203) knots 0 0 0 1 2 2 2
  line L427 (33.8319, 2.7814) -> (30.6979, 2.7814)
  line L428 (30.6979, 2.7814) -> (30.6979, 3.775)
  spline S464 degree 2 poles (30.6979, 3.775) (31.0983, 4.2297) (31.7261, 5.0306) (31.9683, 5.3914) knots 0 0 0 1 2 2 2
  spline S465 degree 2 poles (31.9683, 5.3914) (32.2797, 5.861) (32.5615, 6.5778) (32.5615, 6.9535) knots 0 0 0 1 2 2 2
  spline S466 degree 2 poles (32.5615, 6.9535) (32.5615, 7.3786) (32.2056, 7.8334) (31.8892, 7.8334) knots 0 0 0 1 2 2 2
  spline S467 degree 2 poles (31.8892, 7.8334) (31.7261, 7.8334) (31.4394, 7.7197) (31.2861, 7.6307) knots 0 0 0 1 2 2 2
  spline S468 degree 2 poles (31.2861, 7.6307) (31.1428, 7.5368) (30.9352, 7.3391) (30.8857, 7.2896) knots 0 0 0 1 2 2 2
  line L429 (30.8857, 7.2896) -> (30.8017, 7.2896)
  line L430 (30.8017, 7.2896) -> (30.8017, 8.6194)
  spline S469 degree 2 poles (30.8017, 8.6194) (30.9797, 8.743) (31.7508, 9) (32.1018, 9) knots 0 0 0 1 2 2 2
  spline S470 degree 2 poles (32.1018, 9) (32.863, 9) (33.6441, 8.0311) (33.6441, 7.1562) knots 0 0 0 1 2 2 2
  spline S471 degree 2 poles (33.6441, 7.1562) (33.6441, 6.6173) (33.2882, 5.5793) (32.8779, 4.9861) knots 0 0 0 1 2 2 2
  spline S472 degree 2 poles (32.8779, 4.9861) (32.6208, 4.6203) (32.1314, 4.0518) (32.0227, 3.9331) knots 0 0 0 1 2 2 2
  line L431 (32.0227, 3.9331) -> (33.8319, 3.9331)
  line L432 (33.8319, 3.9331) -> (33.8319, 2.7814)
  line L433 (37.5641, 2.7814) -> (34.4301, 2.7814)
  line L434 (34.4301, 2.7814) -> (34.4301, 3.775)
  spline S473 degree 2 poles (34.4301, 3.775) (34.8305, 4.2297) (35.4583, 5.0306) (35.7005, 5.3914) knots 0 0 0 1 2 2 2
  spline S474 degree 2 poles (35.7005, 5.3914) (36.0119, 5.861) (36.2937, 6.5778) (36.2937, 6.9535) knots 0 0 0 1 2 2 2
  spline S475 degree 2 poles (36.2937, 6.9535) (36.2937, 7.3786) (35.9378, 7.8334) (35.6214, 7.8334) knots 0 0 0 1 2 2 2
  spline S476 degree 2 poles (35.6214, 7.8334) (35.4583, 7.8334) (35.1716, 7.7197) (35.0183, 7.6307) knots 0 0 0 1 2 2 2
  spline S477 degree 2 poles (35.0183, 7.6307) (34.875, 7.5368) (34.6673, 7.3391) (34.6179, 7.2896) knots 0 0 0 1 2 2 2
  line L435 (34.6179, 7.2896) -> (34.5339, 7.2896)
  line L436 (34.5339, 7.2896) -> (34.5339, 8.6194)
  spline S478 degree 2 poles (34.5339, 8.6194) (34.7118, 8.743) (35.483, 9) (35.834, 9) knots 0 0 0 1 2 2 2
  spline S479 degree 2 poles (35.834, 9) (36.5952, 9) (37.3763, 8.0311) (37.3763, 7.1562) knots 0 0 0 1 2 2 2
  spline S480 degree 2 poles (37.3763, 7.1562) (37.3763, 6.6173) (37.0203, 5.5793) (36.61, 4.9861) knots 0 0 0 1 2 2 2
  spline S481 degree 2 poles (36.61, 4.9861) (36.353, 4.6203) (35.8636, 4.0518) (35.7549, 3.9331) knots 0 0 0 1 2 2 2
  line L437 (35.7549, 3.9331) -> (37.5641, 3.9331)
  line L438 (37.5641, 3.9331) -> (37.5641, 2.7814)
  spline S482 degree 2 poles (23.7776, 25.8264) (23.7776, 25.0355) (23.5996, 23.8491) (23.4068, 23.4487) knots 0 0 0 1 2 2 2
  spline S483 degree 2 poles (23.4068, 23.4487) (23.2091, 23.0532) (22.5862, 22.6479) (22.1364, 22.6479) knots 0 0 0 1 2 2 2
  spline S484 degree 2 poles (22.1364, 22.6479) (21.6865, 22.6479) (21.0588, 23.0532) (20.861, 23.4586) knots 0 0 0 1 2 2 2
  spline S485 degree 2 poles (20.861, 23.4586) (20.6682, 23.859) (20.4903, 25.0355) (20.4903, 25.8264) knots 0 0 0 1 2 2 2
  spline S486 degree 2 poles (20.4903, 25.8264) (20.4903, 26.6371) (20.6633, 27.784) (20.866, 28.1992) knots 0 0 0 1 2 2 2
  spline S487 degree 2 poles (20.866, 28.1992) (21.0686, 28.6045) (21.6964, 29) (22.1364, 29) knots 0 0 0 1 2 2 2
  spline S488 degree 2 poles (22.1364, 29) (22.5961, 29) (23.2091, 28.5848) (23.4068, 28.1745) knots 0 0 0 1 2 2 2
  spline S489 degree 2 poles (23.4068, 28.1745) (23.6045, 27.7741) (23.7776, 26.5926) (23.7776, 25.8264) knots 0 0 0 1 2 2 2
  spline S490 degree 2 poles (22.7049, 25.8264) (22.7049, 26.9584) (22.4429, 27.8729) (22.1364, 27.8729) knots 0 0 0 1 2 2 2
  spline S491 degree 2 poles (22.1364, 27.8729) (21.825, 27.8729) (21.563, 26.9584) (21.563, 25.8215) knots 0 0 0 1 2 2 2
  spline S492 degree 2 poles (21.563, 25.8215) (21.563, 24.7043) (21.825, 23.775) (22.1364, 23.775) knots 0 0 0 1 2 2 2
  spline S493 degree 2 poles (22.1364, 23.775) (22.4429, 23.775) (22.7049, 24.7043) (22.7049, 25.8264) knots 0 0 0 1 2 2 2
  spline S494 degree 2 poles (27.4504, 26.1675) (27.4504, 25.3914) (27.1983, 24.0963) (26.9314, 23.6316) knots 0 0 0 1 2 2 2
  spline S495 degree 2 poles (26.9314, 23.6316) (26.6595, 23.162) (25.8438, 22.6578) (25.2506, 22.6578) knots 0 0 0 1 2 2 2
  spline S496 degree 2 poles (25.2506, 22.6578) (25.048, 22.6578) (24.613, 22.7319) (24.5438, 22.7616) knots 0 0 0 1 2 2 2
  line L439 (24.5438, 22.7616) -> (24.5438, 23.9579)
  line L440 (24.5438, 23.9579) -> (24.6278, 23.9579)
  spline S497 degree 2 poles (24.6278, 23.9579) (24.7069, 23.8985) (25.0035, 23.77) (25.2605, 23.77) knots 0 0 0 1 2 2 2
  spline S498 degree 2 poles (25.2605, 23.77) (25.4731, 23.77) (25.8587, 23.9282) (26.002, 24.1012) knots 0 0 0 1 2 2 2
  spline S499 degree 2 poles (26.002, 24.1012) (26.1454, 24.2841) (26.3431, 24.8229) (26.3777, 25.2283) knots 0 0 0 1 2 2 2
  spline S500 degree 2 poles (26.3777, 25.2283) (26.1454, 25.0256) (25.7549, 24.8081) (25.4632, 24.8081) knots 0 0 0 1 2 2 2
  spline S501 degree 2 poles (25.4632, 24.8081) (25.2408, 24.8081) (24.8354, 24.9762) (24.6723, 25.1541) knots 0 0 0 1 2 2 2
  spline S502 degree 2 poles (24.6723, 25.1541) (24.4498, 25.3964) (24.1928, 26.1724) (24.1928, 26.7854) knots 0 0 0 1 2 2 2
  spline S503 degree 2 poles (24.1928, 26.7854) (24.1928, 27.2649) (24.4202, 28.0707) (24.6278, 28.3673) knots 0 0 0 1 2 2 2
  spline S504 degree 2 poles (24.6278, 28.3673) (24.8354, 28.6639) (25.4335, 29) (25.8043, 29) knots 0 0 0 1 2 2 2
  spline S505 degree 2 poles (25.8043, 29) (26.175, 29) (26.7534, 28.7034) (26.961, 28.392) knots 0 0 0 1 2 2 2
  spline S506 degree 2 poles (26.961, 28.392) (27.2032, 28.0459) (27.4504, 26.9485) (27.4504, 26.1675) knots 0 0 0 1 2 2 2
  spline S507 degree 2 poles (26.3925, 26.3949) (26.3925, 26.8942) (26.2739, 27.5368) (26.1701, 27.7147) knots 0 0 0 1 2 2 2
  spline S508 degree 2 poles (26.1701, 27.7147) (26.0959, 27.8482) (25.9081, 27.9619) (25.7994, 27.9619) knots 0 0 0 1 2 2 2
  spline S509 degree 2 poles (25.7994, 27.9619) (25.7054, 27.9619) (25.5275, 27.8532) (25.4434, 27.7147) knots 0 0 0 1 2 2 2
  spline S510 degree 2 poles (25.4434, 27.7147) (25.3693, 27.5961) (25.2655, 27.1364) (25.2655, 26.8645) knots 0 0 0 1 2 2 2
  spline S511 degree 2 poles (25.2655, 26.8645) (25.2655, 26.5679) (25.3693, 26.1873) (25.4632, 26.0736) knots 0 0 0 1 2 2 2
  spline S512 degree 2 poles (25.4632, 26.0736) (25.5522, 25.9599) (25.7895, 25.8709) (25.9328, 25.8709) knots 0 0 0 1 2 2 2
  spline S513 degree 2 poles (25.9328, 25.8709) (26.0515, 25.8709) (26.3085, 25.9648) (26.3827, 26.0143) knots 0 0 0 1 2 2 2
  spline S514 degree 2 poles (26.3827, 26.0143) (26.3827, 26.0588) (26.3925, 26.2268) (26.3925, 26.3949) knots 0 0 0 1 2 2 2
  line L441 (33.6441, 22.7764) -> (30.8264, 22.7764)
  line L442 (30.8264, 22.7764) -> (30.8264, 23.8392)
  line L443 (30.8264, 23.8392) -> (31.7261, 23.8392)
  line L444 (31.7261, 23.8392) -> (31.7261, 27.0672)
  line L445 (31.7261, 27.0672) -> (30.8264, 27.0672)
  line L446 (30.8264, 27.0672) -> (30.8264, 28.0608)
  spline S515 degree 2 poles (30.8264, 28.0608) (31.0241, 28.0608) (31.4147, 28.1349) (31.5333, 28.214) knots 0 0 0 1 2 2 2
  spline S516 degree 2 poles (31.5333, 28.214) (31.6668, 28.3129) (31.82, 28.6441) (31.8299, 28.8912) knots 0 0 0 1 2 2 2
  line L447 (31.8299, 28.8912) -> (32.7642, 28.8912)
  line L448 (32.7642, 28.8912) -> (32.7642, 23.8392)
  line L449 (32.7642, 23.8392) -> (33.6441, 23.8392)
  line L450 (33.6441, 23.8392) -> (33.6441, 22.7764)
  spline S517 degree 2 poles (37.5097, 25.8264) (37.5097, 25.0355) (37.3318, 23.8491) (37.139, 23.4487) knots 0 0 0 1 2 2 2
  spline S518 degree 2 poles (37.139, 23.4487) (36.9412, 23.0532) (36.3184, 22.6479) (35.8686, 22.6479) knots 0 0 0 1 2 2 2
  spline S519 degree 2 poles (35.8686, 22.6479) (35.4187, 22.6479) (34.7909, 23.0532) (34.5932, 23.4586) knots 0 0 0 1 2 2 2
  spline S520 degree 2 poles (34.5932, 23.4586) (34.4004, 23.859) (34.2224, 25.0355) (34.2224, 25.8264) knots 0 0 0 1 2 2 2
  spline S521 degree 2 poles (34.2224, 25.8264) (34.2224, 26.6371) (34.3955, 27.784) (34.5981, 28.1992) knots 0 0 0 1 2 2 2
  spline S522 degree 2 poles (34.5981, 28.1992) (34.8008, 28.6045) (35.4286, 29) (35.8686, 29) knots 0 0 0 1 2 2 2
  spline S523 degree 2 poles (35.8686, 29) (36.3283, 29) (36.9412, 28.5848) (37.139, 28.1745) knots 0 0 0 1 2 2 2
  spline S524 degree 2 poles (37.139, 28.1745) (37.3367, 27.7741) (37.5097, 26.5926) (37.5097, 25.8264) knots 0 0 0 1 2 2 2
  spline S525 degree 2 poles (36.437, 25.8264) (36.437, 26.9584) (36.175, 27.8729) (35.8686, 27.8729) knots 0 0 0 1 2 2 2
  spline S526 degree 2 poles (35.8686, 27.8729) (35.5571, 27.8729) (35.2951, 26.9584) (35.2951, 25.8215) knots 0 0 0 1 2 2 2
  spline S527 degree 2 poles (35.2951, 25.8215) (35.2951, 24.7043) (35.5571, 23.775) (35.8686, 23.775) knots 0 0 0 1 2 2 2
  spline S528 degree 2 poles (35.8686, 23.775) (36.175, 23.775) (36.437, 24.7043) (36.437, 25.8264) knots 0 0 0 1 2 2 2
  line L451 (43.6441, 22.8852) -> (40.8264, 22.8852)
  line L452 (40.8264, 22.8852) -> (40.8264, 23.948)
  line L453 (40.8264, 23.948) -> (41.7261, 23.948)
  line L454 (41.7261, 23.948) -> (41.7261, 27.1759)
  line L455 (41.7261, 27.1759) -> (40.8264, 27.1759)
  line L456 (40.8264, 27.1759) -> (40.8264, 28.1695)
  spline S529 degree 2 poles (40.8264, 28.1695) (41.0241, 28.1695) (41.4147, 28.2437) (41.5333, 28.3228) knots 0 0 0 1 2 2 2
  spline S530 degree 2 poles (41.5333, 28.3228) (41.6668, 28.4216) (41.82, 28.7528) (41.8299, 29) knots 0 0 0 1 2 2 2
  line L457 (41.8299, 29) -> (42.7642, 29)
  line L458 (42.7642, 29) -> (42.7642, 23.948)
  line L459 (42.7642, 23.948) -> (43.6441, 23.948)
  line L460 (43.6441, 23.948) -> (43.6441, 22.8852)
  line L461 (47.3763, 22.8852) -> (44.5586, 22.8852)
  line L462 (44.5586, 22.8852) -> (44.5586, 23.948)
  line L463 (44.5586, 23.948) -> (45.4583, 23.948)
  line L464 (45.4583, 23.948) -> (45.4583, 27.1759)
  line L465 (45.4583, 27.1759) -> (44.5586, 27.1759)
  line L466 (44.5586, 27.1759) -> (44.5586, 28.1695)
  spline S531 degree 2 poles (44.5586, 28.1695) (44.7563, 28.1695) (45.1468, 28.2437) (45.2655, 28.3228) knots 0 0 0 1 2 2 2
  spline S532 degree 2 poles (45.2655, 28.3228) (45.3989, 28.4216) (45.5522, 28.7528) (45.5621, 29) knots 0 0 0 1 2 2 2
  line L467 (45.5621, 29) -> (46.4964, 29)
  line L468 (46.4964, 29) -> (46.4964, 23.948)
  line L469 (46.4964, 23.948) -> (47.3763, 23.948)
  line L470 (47.3763, 23.948) -> (47.3763, 22.8852)
  line L471 (53.6441, 22.7814) -> (50.8264, 22.7814)
  line L472 (50.8264, 22.7814) -> (50.8264, 23.8442)
  line L473 (50.8264, 23.8442) -> (51.7261, 23.8442)
  line L474 (51.7261, 23.8442) -> (51.7261, 27.0721)
  line L475 (51.7261, 27.0721) -> (50.8264, 27.0721)
  line L476 (50.8264, 27.0721) -> (50.8264, 28.0657)
  spline S533 degree 2 poles (50.8264, 28.0657) (51.0241, 28.0657) (51.4147, 28.1399) (51.5333, 28.219) knots 0 0 0 1 2 2 2
  spline S534 degree 2 poles (51.5333, 28.219) (51.6668, 28.3178) (51.82, 28.649) (51.8299, 28.8962) knots 0 0 0 1 2 2 2
  line L477 (51.8299, 28.8962) -> (52.7642, 28.8962)
  line L478 (52.7642, 28.8962) -> (52.7642, 23.8442)
  line L479 (52.7642, 23.8442) -> (53.6441, 23.8442)
  line L480 (53.6441, 23.8442) -> (53.6441, 22.7814)
  line L481 (57.5641, 22.7814) -> (54.4301, 22.7814)
  line L482 (54.4301, 22.7814) -> (54.4301, 23.775)
  spline S535 degree 2 poles (54.4301, 23.775) (54.8305, 24.2297) (55.4583, 25.0306) (55.7005, 25.3914) knots 0 0 0 1 2 2 2
  spline S536 degree 2 poles (55.7005, 25.3914) (56.0119, 25.861) (56.2937, 26.5778) (56.2937, 26.9535) knots 0 0 0 1 2 2 2
  spline S537 degree 2 poles (56.2937, 26.9535) (56.2937, 27.3786) (55.9378, 27.8334) (55.6214, 27.8334) knots 0 0 0 1 2 2 2
  spline S538 degree 2 poles (55.6214, 27.8334) (55.4583, 27.8334) (55.1716, 27.7197) (55.0183, 27.6307) knots 0 0 0 1 2 2 2
  spline S539 degree 2 poles (55.0183, 27.6307) (54.875, 27.5368) (54.6673, 27.3391) (54.6179, 27.2896) knots 0 0 0 1 2 2 2
  line L483 (54.6179, 27.2896) -> (54.5339, 27.2896)
  line L484 (54.5339, 27.2896) -> (54.5339, 28.6194)
  spline S540 degree 2 poles (54.5339, 28.6194) (54.7118, 28.743) (55.483, 29) (55.834, 29) knots 0 0 0 1 2 2 2
  spline S541 degree 2 poles (55.834, 29) (56.5952, 29) (57.3763, 28.0311) (57.3763, 27.1562) knots 0 0 0 1 2 2 2
  spline S542 degree 2 poles (57.3763, 27.1562) (57.3763, 26.6173) (57.0203, 25.5793) (56.61, 24.9861) knots 0 0 0 1 2 2 2
  spline S543 degree 2 poles (56.61, 24.9861) (56.353, 24.6203) (55.8636, 24.0518) (55.7549, 23.9331) knots 0 0 0 1 2 2 2
  line L485 (55.7549, 23.9331) -> (57.5641, 23.9331)
  line L486 (57.5641, 23.9331) -> (57.5641, 22.7814)
  line L487 (13.6441, 12.8852) -> (10.8264, 12.8852)
  line L488 (10.8264, 12.8852) -> (10.8264, 13.948)
  line L489 (10.8264, 13.948) -> (11.7261, 13.948)
  line L490 (11.7261, 13.948) -> (11.7261, 17.1759)
  line L491 (11.7261, 17.1759) -> (10.8264, 17.1759)
  line L492 (10.8264, 17.1759) -> (10.8264, 18.1695)
  spline S544 degree 2 poles (10.8264, 18.1695) (11.0241, 18.1695) (11.4147, 18.2437) (11.5333, 18.3228) knots 0 0 0 1 2 2 2
  spline S545 degree 2 poles (11.5333, 18.3228) (11.6668, 18.4216) (11.82, 18.7528) (11.8299, 19) knots 0 0 0 1 2 2 2
  line L493 (11.8299, 19) -> (12.7642, 19)
  line L494 (12.7642, 19) -> (12.7642, 13.948)
  line L495 (12.7642, 13.948) -> (13.6441, 13.948)
  line L496 (13.6441, 13.948) -> (13.6441, 12.8852)
  line L497 (17.6086, 14.3088) -> (17.0352, 14.3088)
  line L498 (17.0352, 14.3088) -> (17.0352, 12.8703)
  line L499 (17.0352, 12.8703) -> (15.9971, 12.8703)
  line L500 (15.9971, 12.8703) -> (15.9971, 14.3088)
  line L501 (15.9971, 14.3088) -> (14.1285, 14.3088)
  line L502 (14.1285, 14.3088) -> (14.1285, 15.4458)
  line L503 (14.1285, 15.4458) -> (15.9625, 18.9852)
  line L504 (15.9625, 18.9852) -> (17.0352, 18.9852)
  line L505 (17.0352, 18.9852) -> (17.0352, 15.4062)
  line L506 (17.0352, 15.4062) -> (17.6086, 15.4062)
  line L507 (17.6086, 15.4062) -> (17.6086, 14.3088)
  line L508 (15.9971, 15.4062) -> (15.9971, 17.4775)
  line L509 (15.9971, 17.4775) -> (14.9244, 15.4062)
  line L510 (14.9244, 15.4062) -> (15.9971, 15.4062)
  line L511 (13.8319, 2.7764) -> (10.6979, 2.7764)
  line L512 (10.6979, 2.7764) -> (10.6979, 3.77)
  spline S546 degree 2 poles (10.6979, 3.77) (11.0983, 4.2248) (11.7261, 5.0256) (11.9683, 5.3865) knots 0 0 0 1 2 2 2
  spline S547 degree 2 poles (11.9683, 5.3865) (12.2797, 5.8561) (12.5615, 6.5729) (12.5615, 6.9485) knots 0 0 0 1 2 2 2
  spline S548 degree 2 poles (12.5615, 6.9485) (12.5615, 7.3737) (12.2056, 7.8284) (11.8892, 7.8284) knots 0 0 0 1 2 2 2
  spline S549 degree 2 poles (11.8892, 7.8284) (11.7261, 7.8284) (11.4394, 7.7147) (11.2861, 7.6258) knots 0 0 0 1 2 2 2
  spline S550 degree 2 poles (11.2861, 7.6258) (11.1428, 7.5318) (10.9352, 7.3341) (10.8857, 7.2847) knots 0 0 0 1 2 2 2
  line L513 (10.8857, 7.2847) -> (10.8017, 7.2847)
  line L514 (10.8017, 7.2847) -> (10.8017, 8.6144)
  spline S551 degree 2 poles (10.8017, 8.6144) (10.9797, 8.738) (11.7508, 8.9951) (12.1018, 8.9951) knots 0 0 0 1 2 2 2
  spline S552 degree 2 poles (12.1018, 8.9951) (12.863, 8.9951) (13.6441, 8.0262) (13.6441, 7.1512) knots 0 0 0 1 2 2 2
  spline S553 degree 2 poles (13.6441, 7.1512) (13.6441, 6.6124) (13.2882, 5.5743) (12.8779, 4.9811) knots 0 0 0 1 2 2 2
  spline S554 degree 2 poles (12.8779, 4.9811) (12.6208, 4.6153) (12.1314, 4.0468) (12.0227, 3.9282) knots 0 0 0 1 2 2 2
  line L515 (12.0227, 3.9282) -> (13.8319, 3.9282)
  line L516 (13.8319, 3.9282) -> (13.8319, 2.7764)
  spline S555 degree 2 poles (17.5097, 5.8264) (17.5097, 5.0355) (17.3318, 3.8491) (17.139, 3.4487) knots 0 0 0 1 2 2 2
  spline S556 degree 2 poles (17.139, 3.4487) (16.9412, 3.0532) (16.3184, 2.6479) (15.8686, 2.6479) knots 0 0 0 1 2 2 2
  spline S557 degree 2 poles (15.8686, 2.6479) (15.4187, 2.6479) (14.7909, 3.0532) (14.5932, 3.4586) knots 0 0 0 1 2 2 2
  spline S558 degree 2 poles (14.5932, 3.4586) (14.4004, 3.859) (14.2224, 5.0355) (14.2224, 5.8264) knots 0 0 0 1 2 2 2
  spline S559 degree 2 poles (14.2224, 5.8264) (14.2224, 6.6371) (14.3955, 7.784) (14.5981, 8.1992) knots 0 0 0 1 2 2 2
  spline S560 degree 2 poles (14.5981, 8.1992) (14.8008, 8.6045) (15.4286, 9) (15.8686, 9) knots 0 0 0 1 2 2 2
  spline S561 degree 2 poles (15.8686, 9) (16.3283, 9) (16.9412, 8.5848) (17.139, 8.1745) knots 0 0 0 1 2 2 2
  spline S562 degree 2 poles (17.139, 8.1745) (17.3367, 7.7741) (17.5097, 6.5926) (17.5097, 5.8264) knots 0 0 0 1 2 2 2
  spline S563 degree 2 poles (16.437, 5.8264) (16.437, 6.9584) (16.175, 7.8729) (15.8686, 7.8729) knots 0 0 0 1 2 2 2
  spline S564 degree 2 poles (15.8686, 7.8729) (15.5571, 7.8729) (15.2951, 6.9584) (15.2951, 5.8215) knots 0 0 0 1 2 2 2
  spline S565 degree 2 poles (15.2951, 5.8215) (15.2951, 4.7043) (15.5571, 3.775) (15.8686, 3.775) knots 0 0 0 1 2 2 2
  spline S566 degree 2 poles (15.8686, 3.775) (16.175, 3.775) (16.437, 4.7043) (16.437, 5.8264) knots 0 0 0 1 2 2 2
  line L517 (13.8319, -7.2186) -> (10.6979, -7.2186)
  line L518 (10.6979, -7.2186) -> (10.6979, -6.225)
  spline S567 degree 2 poles (10.6979, -6.225) (11.0983, -5.7703) (11.7261, -4.9694) (11.9683, -4.6086) knots 0 0 0 1 2 2 2
  spline S568 degree 2 poles (11.9683, -4.6086) (12.2797, -4.139) (12.5615, -3.4222) (12.5615, -3.0465) knots 0 0 0 1 2 2 2
  spline S569 degree 2 poles (12.5615, -3.0465) (12.5615, -2.6214) (12.2056, -2.1666) (11.8892, -2.1666) knots 0 0 0 1 2 2 2
  spline S570 degree 2 poles (11.8892, -2.1666) (11.7261, -2.1666) (11.4394, -2.2803) (11.2861, -2.3693) knots 0 0 0 1 2 2 2
  spline S571 degree 2 poles (11.2861, -2.3693) (11.1428, -2.4632) (10.9352, -2.6609) (10.8857, -2.7104) knots 0 0 0 1 2 2 2
  line L519 (10.8857, -2.7104) -> (10.8017, -2.7104)
  line L520 (10.8017, -2.7104) -> (10.8017, -1.3806)
  spline S572 degree 2 poles (10.8017, -1.3806) (10.9797, -1.257) (11.7508, -1) (12.1018, -1) knots 0 0 0 1 2 2 2
  spline S573 degree 2 poles (12.1018, -1) (12.863, -1) (13.6441, -1.9689) (13.6441, -2.8438) knots 0 0 0 1 2 2 2
  spline S574 degree 2 poles (13.6441, -2.8438) (13.6441, -3.3827) (13.2882, -4.4207) (12.8779, -5.0139) knots 0 0 0 1 2 2 2
  spline S575 degree 2 poles (12.8779, -5.0139) (12.6208, -5.3797) (12.1314, -5.9482) (12.0227, -6.0669) knots 0 0 0 1 2 2 2
  line L521 (12.0227, -6.0669) -> (13.8319, -6.0669)
  line L522 (13.8319, -6.0669) -> (13.8319, -7.2186)
  spline S576 degree 2 poles (17.5394, -5.1425) (17.5394, -6.1064) (16.6842, -7.3472) (15.9427, -7.3472) knots 0 0 0 1 2 2 2
  spline S577 degree 2 poles (15.9427, -7.3472) (15.572, -7.3472) (14.9837, -7.0407) (14.781, -6.7391) knots 0 0 0 1 2 2 2
  spline S578 degree 2 poles (14.781, -6.7391) (14.5388, -6.3882) (14.2818, -5.2759) (14.2818, -4.4998) knots 0 0 0 1 2 2 2
  spline S579 degree 2 poles (14.2818, -4.4998) (14.2818, -3.699) (14.524, -2.4533) (14.7959, -1.9738) knots 0 0 0 1 2 2 2
  spline S580 degree 2 poles (14.7959, -1.9738) (15.0529, -1.519) (15.8982, -1.0049) (16.4716, -1.0049) knots 0 0 0 1 2 2 2
  spline S581 degree 2 poles (16.4716, -1.0049) (16.6793, -1.0049) (17.0994, -1.084) (17.1785, -1.1088) knots 0 0 0 1 2 2 2
  line L523 (17.1785, -1.1088) -> (17.1785, -2.305)
  line L524 (17.1785, -2.305) -> (17.0994, -2.305)
  spline S582 degree 2 poles (17.0994, -2.305) (17.0253, -2.2506) (16.6842, -2.1172) (16.4618, -2.1172) knots 0 0 0 1 2 2 2
  spline S583 degree 2 poles (16.4618, -2.1172) (15.9625, -2.1172) (15.4187, -2.8735) (15.3545, -3.5754) knots 0 0 0 1 2 2 2
  spline S584 degree 2 poles (15.3545, -3.5754) (15.567, -3.3827) (15.9971, -3.1553) (16.269, -3.1553) knots 0 0 0 1 2 2 2
  spline S585 degree 2 poles (16.269, -3.1553) (16.4964, -3.1553) (16.9017, -3.3332) (17.0599, -3.5013) knots 0 0 0 1 2 2 2
  spline S586 degree 2 poles (17.0599, -3.5013) (17.2774, -3.7435) (17.5394, -4.5295) (17.5394, -5.1425) knots 0 0 0 1 2 2 2
  spline S587 degree 2 poles (16.2937, -6.0619) (16.3777, -5.9136) (16.4667, -5.5676) (16.4667, -5.2166) knots 0 0 0 1 2 2 2
  spline S588 degree 2 poles (16.4667, -5.2166) (16.4667, -4.92) (16.3629, -4.5344) (16.269, -4.4207) knots 0 0 0 1 2 2 2
  spline S589 degree 2 poles (16.269, -4.4207) (16.175, -4.3021) (15.9378, -4.2181) (15.7994, -4.2181) knots 0 0 0 1 2 2 2
  spline S590 degree 2 poles (15.7994, -4.2181) (15.6906, -4.2181) (15.4533, -4.3021) (15.3495, -4.3614) knots 0 0 0 1 2 2 2
  spline S591 degree 2 poles (15.3495, -4.3614) (15.3495, -4.401) (15.3446, -4.5888) (15.3446, -4.7322) knots 0 0 0 1 2 2 2
  spline S592 degree 2 poles (15.3446, -4.7322) (15.3446, -5.2611) (15.4731, -5.8988) (15.572, -6.0619) knots 0 0 0 1 2 2 2
  spline S593 degree 2 poles (15.572, -6.0619) (15.6461, -6.1954) (15.834, -6.3091) (15.9427, -6.3091) knots 0 0 0 1 2 2 2
  spline S594 degree 2 poles (15.9427, -6.3091) (16.0267, -6.3091) (16.2245, -6.1855) (16.2937, -6.0619) knots 0 0 0 1 2 2 2
  dimension "d20" = 6
  dimension "d21" = 5
  dimension "d22" = 1
  dimension "d23" = 1.5
  dimension "d24" = 6
  dimension "d25" = 5
  dimension "d26" = 1
  dimension "d27" = 1.5
  dimension "d28" = 6
  dimension "d29" = 5
  dimension "d30" = 1
  dimension "d31" = 1.5
  dimension "d32" = 6
  dimension "d33" = 5
  dimension "d34" = 1
  dimension "d35" = 1.5
  dimension "d36" = 5
  dimension "d37" = 6
  dimension "d38" = 1
  dimension "d39" = 1.5
  dimension "d40" = 5
  dimension "d41" = 6
  dimension "d42" = 1
  dimension "d43" = 1.5
  dimension "d44" = 5
  dimension "d45" = 6
  dimension "d46" = 1
  dimension "d47" = 1.5
  dimension "d48" = 6
  dimension "d49" = 5
  dimension "d50" = 1
  dimension "d51" = 1.5
  dimension "d52" = 6
  dimension "d53" = 5
  dimension "d54" = 1
  dimension "d55" = 1.5
  dimension "d56" = 6
  dimension "d57" = 7